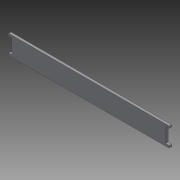
# Autodesk Inventor part: Fin
Saved by Autodesk Inventor 2015 (Build 190159000, 159)
## iProperties
Created: 2014-07-01
Part Number: Fin
Material: Generic
Document SubType Name: Modeling
Designer: STACKPOLE
Density: 1 g/cm^3
Appearance: Default
Author: STACKPOLE
Autodesk Inventor part; units mm, degrees
ref_plane "YZ Plane" through (0, 0, 0) normal (1, 0, 0) x (0, 1, 0)
ref_plane "XZ Plane" through (0, 0, 0) normal (0, 1, 0) x (-1, 0, 0)
ref_plane "XY Plane" through (0, 0, 0) normal (0, 0, 1) x (1, 0, 0)
sketch "Sketch1" plane through (0, 0, 0) normal (0, 1, 0) x (-1, 0, 0)
  line L0 (0, 1) -> (0, 2)
  line L1 (1, 3) -> (5, 3)
  line L2 (5, 22) -> (1, 22)
  line L3 (0, 23) -> (0, 24)
  line L4 (1, 25) -> (105, 25)
  line L5 (105, 25) -> (105, 0) construction
  line L6 (105, 0) -> (1, 0)
  line L7 (5, 3) -> (5, 22)
  arc A0 (1, 25) -> (0, 24) centre (1, 24) ccw
  arc A1 (0, 23) -> (1, 22) centre (1, 23) ccw
  arc A2 (1, 3) -> (0, 2) centre (1, 2) ccw
  arc A3 (0, 1) -> (1, 0) centre (1, 1) ccw
  line L8 (210, 1) -> (210, 2)
  line L9 (209, 3) -> (205, 3)
  line L10 (205, 22) -> (209, 22)
  line L11 (210, 23) -> (210, 24)
  line L12 (209, 25) -> (105, 25)
  line L13 (105, 0) -> (209, 0)
  line L14 (196.5, 16) -> (105, 16) construction
  line L15 (205, 3) -> (205, 22)
  arc A4 (210, 24) -> (209, 25) centre (209, 24) ccw
  arc A5 (209, 22) -> (210, 23) centre (209, 23) ccw
  arc A6 (210, 2) -> (209, 3) centre (209, 2) ccw
  arc A7 (209, 0) -> (210, 1) centre (209, 1) ccw
  point P0 (0, 0)
  point P1 (0, 3)
  point P2 (0, 22)
  point P3 (0, 25)
  point P4 (210, 0)
  point P5 (210, 3)
  point P6 (210, 22)
  point P7 (210, 25)
  dimension "d0" = 3
  dimension "d1" = 5
  dimension "d3" = 3
  dimension "d4" = 105
  dimension "d5" = 5
  dimension "d15" = 1
  dimension "d18" = 25
  constraints: 32 end point, 19 symmetric about line, 17 point on line, 16 point on circle, 8 centre point, 8 tangent, 5 parallel, 3 equal radius, 1 collinear, 1 perpendicular, 1 vertical, 4 other
  measures "d0" distance of point (0, 0) point (0, 3)
  measures "d1" distance of point (0, 3) L1.end
  measures "d3" distance of point (0, 22) point (0, 25)
  measures "d4" distance of point (0, 25) L4.end
  measures "d5" distance of L2.start point (0, 22)
  measures "d15" radius of A0
  measures "d18" distance between parallel lines of L6 L4
extrude "Extrusion1" add sketch "Sketch1" along normal blind 3
body "Solid1"
